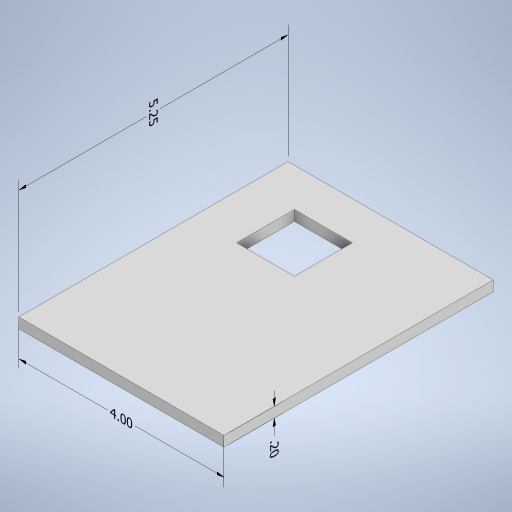
# Autodesk Inventor part: HalfofTop
Saved by Autodesk Inventor 2024.3 (Build 283343010, 343A)
## iProperties
Created: 2025-04-11
Part Number: HalfofTop
Material: Generic
Document SubType Name: Modeling
Designer: Vincent Larson
Density: 1 g/cm^3
Appearance: Default
Author: Vincent Larson
Autodesk Inventor part; units mm, degrees
ref_plane "YZ Plane" through (0, 0, 0) normal (1, 0, 0) x (0, 1, 0)
ref_plane "XZ Plane" through (0, 0, 0) normal (0, 1, 0) x (-1, 0, 0)
ref_plane "XY Plane" through (0, 0, 0) normal (0, 0, 1) x (1, 0, 0)
sketch "Sketch1" plane through (0, 0, 0) normal (0, 1, 0) x (-1, 0, 0)
  line L0 (0, 0) -> (-101.6, 0)
  line L1 (-101.6, 0) -> (-101.6, -133.35)
  line L2 (-101.6, -133.35) -> (0, -133.35)
  line L3 (0, -133.35) -> (0, 0)
  dimension "d0" = 101.6
  dimension "d1" = 133.35
  constraints: 8 end point, 2 parallel, 1 horizontal, 1 perpendicular
  measures "d0" distance of L2.end L1.end
  measures "d1" distance of L1.end L0.end
extrude "Extrusion1" add sketch "Sketch1" along normal blind 5.08
sketch "Sketch2" plane through (0, 5.08, 0) normal (0, 1, 0) x (1, 0, 0)
  line L0 (101.6, 133.35) -> (0, 133.35) projected
  line L1 (50.8, 133.35) -> (50.8, 114.3)
  line L2 (50.8, 114.3) -> (22.225, 114.3)
  line L3 (22.225, 114.3) -> (22.225, 85.725)
  line L4 (22.225, 85.725) -> (50.8, 85.725)
  line L5 (50.8, 85.725) -> (50.8, 114.3)
  point P0 (0, 0)
  dimension "d4" = 19.05
  dimension "d5" = 28.575
  dimension "d6" = 28.575
  constraints: 10 end point, 2 parallel, 1 horizontal, 1 midpoint, 1 perpendicular, 1 vertical
  measures "d4" distance of L1.start L1.end
  measures "d5" distance of L4.end L3.end
  measures "d6" distance of L3.end L2.end
extrude "Extrusion2" cut sketch "Sketch2" against normal blind 25.4
body "Solid1"
